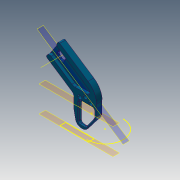
# Autodesk Inventor part: J005483
Saved by Autodesk Inventor 2015 SP1 (Build 190203100, 203)
## iProperties
Created: 2014-10-29
Material: TITANIUM, 6AL-4V, ANNEALED
Vendor: HHMI: JRC - ID&F
Document SubType Name: Sheet Metal
Designer: arnoldj
Density: 4.43 g/cm^3
Sheet Metal Rule: Default
Description: MBS INLINE D TAB
Mass: 1.83252 g
Surface Area: 7.44075 cm^2
Volume: 0.41366 cm^3
Project: P-243001
Appearance: Sky Blue Dark
Part Number: J005483
RuleStatus: InUse
AfterDocSave0: file://Part Number Cleaner
DESIGN DEPARTMENT: HHMI: JRC - ID&F
SPECIAL FINISH: NONE
LAB/DEPT: SVOBODA (LAB)
REQUESTING SCIENTIST: SOFRONIEW, NICK
SURFACE ROUGHNESS: 63 Ra
Thickness: 0.100 in
ALTERED ITEM PART NUMBER: N/A
ALTERED ITEM VENDOR: N/A
ALTERED ITEM DESCRIPTION: N/A
Revision Number: A
Autodesk Inventor part; units mm, degrees
ref_plane "YZ Plane" through (0, 0, 0) normal (1, 0, 0) x (0, 1, 0)
sketch "Sketch1" plane through (0, 0, 0) normal (0, 0, 1) x (1, 0, 0)
  line L0 (-3.048, -0.6985) -> (-3.048, 17.064)
  line L1 (6.9036, 2.286) -> (6.9036, 10.4772)
  line L2 (-3.048, -1.143) -> (-3.048, -1.143) construction
  line L3 (-1.397, -6.35) -> (-1.905, -6.35)
  line L4 (-3.048, 5.0324) -> (-15.3447, 13.1713)
  line L5 (-15.3447, 13.1713) -> (-9.8071, 21.5377)
  line L6 (-9.8071, 21.5377) -> (6.9036, 10.4772)
  line L7 (-15.3447, 13.1713) -> (-28.0607, 13.1713) construction
  line L8 (-12.5759, 17.3545) -> (0, 9.0307) construction
  line L9 (-9.5394, 13.0603) -> (-7.4366, 16.2374)
  line L10 (-7.4366, 16.2374) -> (-10.1053, 18.0038)
  line L11 (-10.1053, 18.0038) -> (-12.2082, 14.8267)
  line L12 (-12.2082, 14.8267) -> (-9.5394, 13.0603)
  line L13 (-9.5394, 13.0603) -> (-10.1053, 18.0038) construction
  line L14 (-7.4366, 16.2374) -> (-12.2082, 14.8267) construction
  line L15 (0, 27.8773) -> (0, -16.4995) projected
  line L16 (-38.7577, 0) -> (36.1216, 0) projected
  line L17 (6.9036, 2.286) -> (6.9036, 0.3427)
  line L18 (6.9036, 0.3427) -> (2.1297, -6.35)
  line L19 (2.1297, -6.35) -> (-1.397, -6.35)
  line L20 (5.7606, 3.7609) -> (5.7606, 0.0525)
  line L21 (5.7606, 0.0525) -> (2.2808, -4.826)
  line L22 (2.2808, -4.826) -> (-0.9196, -4.826)
  line L23 (-0.9196, 3.7609) -> (-0.9196, -4.826)
  line L24 (-0.9196, 3.7609) -> (5.7606, 3.7609)
  line L25 (-9.8071, 21.5377) -> (25.4246, 21.5377) construction
  line L26 (-3.048, -0.6985) -> (-1.905, -6.35)
  point P0 (0, 0)
  point P1 (0, 0)
  point P2 (0, 0)
  point P3 (0, 0)
  point P4 (2.103, -1.214)
  point P5 (-9.8224, 15.532)
  dimension "d161" = 123.5
  dimension "d162" = 10.033
  dimension "d177" = 146.5
  dimension "d180" = 9.0307
  dimension "d210" = 4.8006
  dimension "d221" = 3.302
  dimension "d232" = 3.2004
  dimension "d233" = 3.81
  dimension "d262" = 1.214
  dimension "d264" = 16.746
  dimension "d270" = 1.524
  dimension "d271" = 1.143
  dimension "d283" = 9.9516
  dimension "d296" = 144.5
  dimension "d297" = 6.35
  dimension "d298" = 6.6802
  dimension "d299" = 3.2004
  dimension "d342" = 27.8877
  dimension "d370" = 2.103
  dimension "d371" = 3.048
  dimension "d373" = 8.5869
  dimension "d374" = 3.7084
  dimension "d377" = 0.762
  dimension "d384" = 5.6515
  dimension "d385" = 1.143
  dimension "d394" = 9.8224
  constraints: 50 end point, 6 perpendicular, 5 parallel, 5 point on line, 5 vertical, 3 horizontal, 3 midpoint, 2 coincident
  measures "d161" angle of L4 L0
  measures "d162" distance of L4.end L5.end
  measures "d177" angle of L4 L7
  measures "d180" distance of L8.end point (0, 0)
  measures "d210" distance from line of L1 point (2.103, -1.214)
  measures "d221" distance from line of point (-9.822, 15.532) L5
  measures "d232" distance of L9.end L10.end
  measures "d233" distance of L9.start L9.end
  measures "d262" distance from line of L16 point (2.103, -1.214)
  measures "d264" vertical distance of point (2.103, -1.214) point (-9.822, 15.532)
  measures "d270" distance between parallel lines of L19 L22
  measures "d271" distance between parallel lines of L17 L20
  measures "d283" distance between parallel lines of L17 L0
  measures "d296" angle of L21 L20
  measures "d297" distance between parallel lines of L16 L3
  measures "d298" distance of L23.start L20.start
  measures "d299" distance of L21.end L22.end
  measures "d342" distance between parallel lines of L19 L25
  measures "d370" distance from line of point (2.103, -1.214) L15
  measures "d371" distance between parallel lines of L0 L15
  measures "d373" distance of L23.start L22.end
  measures "d374" distance of L20.start L20.end
  measures "d377" distance between parallel lines of L18 L21
  measures "d384" distance from line of L0.start L3
  measures "d385" distance from line of L3.end L0
  measures "d394" distance from line of L15 point (-9.822, 15.532)
ref_plane "Work Plane1" through (0, 10.16, 0) normal (0, 1, 0) x (-1, 0, 0)
extrude "Plate1" add sketch "Sketch1" along normal blind 2.54 contours L4 L5 L6 L0 | L0 L6 L15 L24 L23 L16 | L16 L23 L22 L15 L19 L3 L26 L0 | L6 L1 L17 L18 L16 L21 L20 L24 L15 | L22 L21 L16 L18 L19 L15
sketch "Sketch7" plane through (0, 0, 0) normal (0, 0, 1) x (1, 0, 0)
  circle A0 centre (1.9278, 6.3009) radius 0.8255
  circle A1 centre (-0.508, 5.0309) radius 0.8255
  circle A2 centre (4.3636, 5.0309) radius 0.8255
  line L0 (0, 23.5626) -> (0, -15.7804) construction
  circle A3 centre (0, 7.5709) radius 0.8255
  circle A4 centre (3.8556, 7.5709) radius 0.8255
  circle A5 centre (-2.9516, 0.722) radius 0.8255
  line L1 (-3.048, -6.35) -> (-3.048, 5.0324) projected
  line L2 (-2.8229, -6.3894) -> (-3.048, -1.143) construction
  line L3 (-22.6717, 0) -> (18.6824, 0) projected
  line L4 (6.9036, 10.4772) -> (6.9036, 0.3427) projected
  line L5 (1.75, 2.286) -> (1.75, -2.667) construction
  line L6 (-0.508, 5.0309) -> (4.3636, 5.0309) construction
  line L7 (0, 7.5709) -> (3.8556, 7.5709) construction
  line L8 (1.9278, 7.5709) -> (1.9278, 5.0309) construction
  line L9 (-0.9196, 3.7609) -> (5.7606, 3.7609) projected
  point P0 (0, 0)
  point P1 (-3.048, -1.143)
  point P2 (-1.905, -6.35)
  point P3 (-3.048, 17.064)
  dimension "d61" = 1.651
  dimension "d252" = 2.54
  dimension "d255" = 3.048
  dimension "d259" = 9.8552
  dimension "d273" = 0.0964
  dimension "d275" = 3.048
  dimension "d281" = 2.54
  dimension "d375" = 2.54
  dimension "d376" = 1.27
  constraints: 8 end point, 6 centre point, 5 equal radius, 3 coincident, 3 midpoint, 1 horizontal, 1 vertical, 2 other
  measures "d61" diameter of A0
  measures "d252" distance from line of L4 L6.end
  measures "d255" distance from line of point (3.856, 7.571) L4
  measures "d259" distance from line of A5.centre L4
  measures "d375" distance between parallel lines of L7 L6
  measures "d376" distance between parallel lines of L9 L6
hole "Hole2" at (-0.508, 5.0309, 0) at (4.3636, 5.0309, 0) at (1.9278, 6.3009, 0) direction (0, 0, 1) diameter 1.651 depth 2.54 tip angle 118
ref_plane "Work Plane3" through (0, 0, 1.143) normal (0, 0, 1) x (1, 0, 0)
fillet "Fillet8" radius 8.255 1 edges at (6.9036, 10.4772, 1.27)
sketch "Sketch9" plane through (0, 0, 0) normal (0, 0, 1) x (1, 0, 0)
  point P0 (0, 0)
sketch "Sketch10" plane through (0, 0, 0) normal (0, 0, 1) x (1, 0, 0)
  circle A0 centre (2.6461, -1.2506) radius 3.5
  point P0 (0, 0)
  dimension "d150" = 7
  constraints: 1 centre point
  measures "d150" diameter of A0
sketch "Sketch3" plane through (0, 0, 2.54) normal (0, 0, 1) x (1, 0, 0)
  line L0 (-16.764, 14.16) -> (4.445, 14.16)
  line L1 (-4.445, 6.16) -> (-16.764, 6.16)
  line L2 (-6.35, 14.16) -> (-6.35, 6.16)
  line L3 (0, 17.9421) -> (0, -8.5328)
  line L4 (12.7747, 8.2785) -> (4.445, 8.2785)
  point P0 (0, 0)
  point P1 (-5.2531, 14.0148)
  point P2 (4.445, 14.16)
  dimension "d15" = 6.35
  constraints: 8 end point, 1 perpendicular, 1 point on line, 4 other
  measures "d15" distance between parallel lines of L3 L2
fillet "Fillet15" radius 0.762 4 edges at (5.7606, 0.0525, 1.27) (2.2808, -4.826, 1.27) (-0.9196, 3.7609, 1.27) (-0.9196, -4.826, 1.27)
fillet "Fillet7" radius 2.54 2 edges at (2.1297, -6.35, 1.27) (6.9036, 0.3427, 1.27)
sketch "Sketch15" plane through (0, 0, 0) normal (0, 0, 1) x (1, 0, 0)
  point P0 (0, 0)
fillet "Fillet19" radius 1.27 4 edges at (-10.1053, 18.0038, 1.27) (-7.4366, 16.2374, 1.27) (-9.5394, 13.0603, 1.27) (-12.2082, 14.8267, 1.27)
fillet "Fillet20" radius 0.635 2 edges at (-15.3447, 13.1713, 1.27) (-9.8071, 21.5377, 1.27)
fillet "Fillet21" radius 1.905 1 edges at (-3.048, 5.0324, 1.27)
sketch "Sketch18" plane through (0, 0, 2.54) normal (0, 0, 1) x (1, 0, 0)
  line L0 (-10.1576, 21.0082) -> (-14.9942, 13.7009) projected
  line L1 (-14.118, 15.0246) -> (-11.0338, 19.6844)
  line L2 (-11.0338, 19.6844) -> (-2.5615, 14.0767)
  line L3 (-2.5615, 14.0767) -> (-5.6457, 9.417)
  line L4 (-5.6457, 9.417) -> (-14.118, 15.0246)
  line L5 (-12.5759, 17.3545) -> (-4.1036, 11.7468) construction
  line L6 (-12.5759, 17.3545) -> (0.4236, 8.7504) construction
  line L7 (-14.9942, 13.7009) -> (-10.1576, 21.0082) construction
  line L8 (-9.2776, 21.1872) -> (3.2048, 12.9253) construction
  line L9 (-3.9016, 5.5973) -> (-14.8151, 12.8209) projected
  line L10 (3.5097, 10.0583) -> (-2.5615, 14.0767)
  line L11 (-5.6457, 9.417) -> (-3.3158, 7.8749)
  line L12 (-3.3158, 7.8749) -> (2.8525, 7.8749)
  circle A0 centre (2.8525, 9.0655) radius 1.1906
  point P0 (0, 0)
  point P1 (-3.048, 17.064)
  dimension "d315" = 5.588
  dimension "d318" = 10.16
  dimension "d319" = 2.2225
  dimension "d355" = 2.3813
  dimension "d356" = 2.794
  constraints: 18 end point, 4 midpoint, 2 collinear, 2 parallel, 2 point on circle, 2 point on line, 2 tangent, 1 centre point, 1 horizontal, 1 perpendicular
  measures "d315" distance between parallel lines of L4 L2
  measures "d318" distance of L1.end L2.end
  measures "d319" distance between parallel lines of L2 L8
  measures "d355" diameter of A0
  measures "d356" distance of L3.end L11.end
extrude "Extrusion10" cut sketch "Sketch18" against normal blind 1.27
fillet "Fillet24" radius 2.3813 1 edges at (-3.3158, 7.8749, 1.905)
fillet "Fillet25" radius 1.27 2 edges at (-11.0338, 19.6844, 1.905) (-14.118, 15.0246, 1.905)
chamfer "Chamfer7" distance 0.254 angle 45 16 edges at (-10.0004, 17.4883, 1.27) (-11.1568, 16.4152, 1.27) (-11.6927, 14.9316, 1.27) (-10.8738, 13.9435, 1.27) (-9.6443, 13.5758, 1.27) (-8.488, 14.6488, 1.27) (-7.952, 16.1325, 1.27) (-8.7709, 17.1206, 1.27) (-10.0004, 17.4883, 0) (-8.7709, 17.1206, 0) (-7.952, 16.1325, 0) (-8.488, 14.6488, 0) (-9.6443, 13.5758, 0) (-10.8738, 13.9435, 0) (-11.6927, 14.9316, 0) (-11.1568, 16.4152, 0)
fillet "Fillet28" radius 0.762 1 edges at (5.7606, 3.7609, 1.27)
ref_plane "Work Plane8" through (0, 1.27, 0) normal (0, 1, 0) x (-1, 0, 0)
ref_plane "Work Plane10" through (0, -10.16, 0) normal (0, 1, 0) x (-1, 0, 0)
sketch "Sketch20" plane through (0, 0, 0) normal (0, 1, 0) x (-1, 0, 0)
  circle A0 centre (-2.032, -6.0325) radius 7.9375
  line L0 (0, -17.272) -> (0, 5.842) projected
  line L1 (-18.6824, 0) -> (22.6717, 0) projected
  point P0 (0, 0)
  dimension "d344" = 15.875
  dimension "d345" = 2.032
  dimension "d346" = 6.0325
  constraints: 1 centre point
  measures "d344" diameter of A0
  measures "d345" distance from line of A0.centre L0
  measures "d346" distance from line of L1 A0.centre
extrude "Extrusion12" cut sketch "Sketch20" against normal up to surface (11.43 mm away) from surface at 1.27
sketch "Sketch21" plane through (0, 1.27, 0) normal (0, 1, 0) x (-1, 0, 0)
  line L0 (0, -19.394) -> (0, 18.5742) projected
  line L1 (-18.6824, 0) -> (22.6717, 0) projected
  arc A0 (-2.032, 1.905) -> (-2.032, -13.97) centre (-2.032, -6.0325) ccw
  line L2 (-2.032, -6.0325) -> (-2.032, 13.1501)
  line L3 (-2.032, 1.905) -> (-2.032, -13.97)
  point P0 (0, 0)
  dimension "d350" = 15.875
  dimension "d351" = 2.032
  dimension "d352" = 6.0325
  constraints: 4 end point, 2 point on circle, 2 point on line, 1 centre point, 1 vertical
  measures "d350" diameter of A0
  measures "d351" distance from line of L2.start L0
  measures "d352" distance from line of L2.start L1
revolve "Revolution1" cut sketch "Sketch21" angle 360 about axis through (2.032, 1.27, -6.0325) along (0, 0, 1)
ref_plane "Work Plane9" through (-9.547, 15.3498, 0.254) normal (-0.551937, -0.8338858, 0) x (0.8338858, -0.551937, 0)
sketch "Sketch22" plane through (0, -10.16, 0) normal (0, 1, 0) x (-1, 0, 0)
  line L0 (0, -18.8738) -> (0, 6.109) projected
  line L1 (-18.6824, 0) -> (22.6717, 0) projected
  arc A0 (-2.032, 1.905) -> (-2.032, -13.97) centre (-2.032, -6.0325) ccw
  line L2 (-2.032, -6.0325) -> (-2.032, -15.3048)
  line L3 (-2.032, -13.97) -> (-2.032, 1.905)
  line L4 (-2.8525, 1.27) -> (2.5991, 1.27) projected
  arc A1 (3.048, 0.0665) -> (0.9196, 1.3358) centre (-2.032, -6.0325) ccw projected
  point P0 (0, 0)
  point P1 (1.0895, 1.0814)
  point P2 (2.814, 0)
  point P3 (3.0986, 0.039)
  point P4 (-6.878, 0)
  dimension "d359" = 15.875
  dimension "d360" = 6.0325
  dimension "d365" = 0
  constraints: 4 end point, 2 point on circle, 1 centre point, 1 perpendicular, 1 point on line, 1 vertical, 1 other
  measures "d359" diameter of A0
  measures "d360" distance from line of L1 L2.start
  measures "d365" horizontal distance of point (-2.032, -6.032) L3.end
sketch "Sketch23" plane through (0, -10.16, 0) normal (0, 1, 0) x (-1, 0, 0)
  arc A0 (-2.032, 1.905) -> (-2.032, -13.97) centre (-2.032, -6.0325) ccw projected
  line L0 (9.2776, 2.54) -> (-3.2048, 2.54) projected
  line L1 (-3.2048, 0) -> (-3.2048, 2.54) projected
  line L2 (-3.2048, 0) -> (9.2776, 0) projected
  line L3 (9.2776, 2.54) -> (9.2776, 0) projected
  point P0 (0, 0)
revolve "Revolution2" [suppressed]
chamfer "Chamfer9" distance 0.381 angle 45 10 edges at (2.4205, 3.7609, 2.54) (5.5374, 3.5377, 2.54) (5.7606, 1.6477, 2.54) (5.7243, 0.0641, 2.54) (4.0638, -2.3263, 2.54) (2.2372, -4.7414, 2.54) (0.8654, -4.826, 2.54) (-0.6964, -4.6028, 2.54) (-0.9196, -0.5326, 2.54) (-0.6964, 3.5377, 2.54)
chamfer "Chamfer10" [suppressed]
fillet "Fillet31" [suppressed]
fillet "Fillet32" radius 2.54 1 edges at (-1.905, -6.35, 1.6999)
sketch "Sketch25" plane through (0, 0, 0) normal (0, 0, 1) x (1, 0, 0)
  line L0 (-22.6717, 1.27) -> (18.6824, 1.27) projected
  arc A0 (4.3949, 5.8558) -> (2.7496, 6.3786) centre (2.032, 1.27) ccw projected
  circle A1 centre (2.032, 1.27) radius 6.6675
  line L1 (-4.6355, -6.985) -> (8.6995, -6.985)
  line L2 (8.6995, -6.985) -> (8.6995, 1.27)
  line L3 (8.6995, 1.27) -> (-4.6355, 1.27)
  line L4 (-4.6355, 1.27) -> (-4.6355, -6.985)
  line L5 (-4.6355, -6.985) -> (8.6995, 1.27) construction
  line L6 (8.6995, -6.985) -> (-4.6355, 1.27) construction
  point P0 (0, 0)
  point P1 (2.032, -2.8575)
  dimension "d386" = 13.335
  dimension "d387" = 8.255
  constraints: 12 end point, 2 midpoint, 2 parallel, 1 coincident, 1 horizontal, 1 horizontal alignment, 1 perpendicular, 1 point on line, 2 other
  measures "d387" distance of L1.end L2.end
extrude "Extrusion13" cut sketch "Sketch25" along normal blind 0.254
fillet "Fillet33" radius 0.381 2 edges at (-3.4087, 5.1242, 0.127) (6.9036, 5.8223, 0.127)
equation "\"d71\" = Thickness"
equation "\"BendRadius\" = Thickness"
equation "\"BendReliefWidth\" = Thickness"
equation "\"BendReliefDepth\" = 0.5 * Thickness"
equation "\"CornerReliefSize\" = 4 * Thickness"
equation "\"MinimumRemnant\" = 2 * Thickness"
equation "\"TransitionRadius\" = BendRadius"
equation "\"JacobiRadiusSize\" = BendRadius"
equation "\"GapSize\" = Thickness"
equation "\"d6\" = BendRadius"
equation "\"Thickness\" = 2.54"
body "Solid1"
